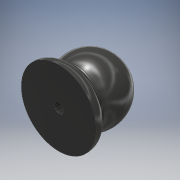
# Autodesk Inventor part: Puxador
Saved by Autodesk Inventor 2018 (Build 220112000, 112)
## iProperties
Created: 2018-07-12
Part Number: Puxador
Material: Plástico PC/ABS
Document SubType Name: Modeling
Designer: Regner
Density: 0.357273 g/cm^3
Appearance: Cinza escuro
Author: Regner
Autodesk Inventor part; units mm, degrees
ref_plane "YZ Plane" through (0, 0, 0) normal (1, 0, 0) x (0, 1, 0)
ref_plane "XZ Plane" through (0, 0, 0) normal (0, 1, 0) x (-1, 0, 0)
ref_plane "XY Plane" through (0, 0, 0) normal (0, 0, 1) x (1, 0, 0)
sketch "Esboço1" plane through (0, 0, 0) normal (0, 1, 0) x (-1, 0, 0)
  circle A0 centre (0, 0) radius 9
  dimension "d0" = 18
  constraints: 1 centre point, 1 coincident
  measures "d0" diameter of A0
extrude "Extrusão1" add sketch "Esboço1" along normal blind 3
fillet "Arredondamento1" radius 2.5 1 edges at (9, 3, 0)
sketch "Esboço2" plane through (0, 0, 0) normal (1, 0, 0) x (0, 1, 0)
  line L0 (3, 6.5) -> (3, -6.5) projected
  line L1 (0, 0) -> (13.7463, 0)
  arc A0 (15, 0) -> (0, 0) centre (7.5, 0) ccw
  line L2 (0, 9) -> (0, -9) projected
  line L3 (15, 0) -> (0, 0)
  dimension "d4" = 15
  constraints: 4 end point, 2 point on circle, 2 point on line, 1 centre point, 1 horizontal, 1 perpendicular, 1 tangent
  measures "d4" diameter of A0
revolve "Revolução1" add sketch "Esboço2" angle 360 about axis through (0, 0, 0) along (0, 1, 0)
fillet "Arredondamento2" radius 1 1 edges at (0, 3, -6)
hole "Furo1" at (0, 0, 0) direction (0, 1, 0) diameter 2.4 depth 8 clearance for "Countersunk Flat Head Screw ISO 2009/7046" size "M2" standard "ISO"
